rear_ear_v2_heatset (Autodesk Fusion 360 design; units mm, degrees)
part number: 2025-11-01-16-26-23-759
Autodesk Fusion 360 part; units mm, degrees
note: some values were not read from the file. Chosen so that the rebuilt part matches the saved one: a direction; which bodies a step acts on. Set by a fixed rule: which sketch regions a step uses.
sketch "Sketch1" plane through (0, 0, 0) normal (0, 0, 1) x (1, 0, 0)
  line L0 (0, 0) -> (15.875, 0)
  line L1 (15.875, 0) -> (15.875, 44.45)
  line L2 (15.875, 44.45) -> (0, 44.45)
  line L3 (0, 44.45) -> (0, 0)
  circle A0 centre (7.9375, 6.35) radius 2.4
  line L4 (7.9375, 44.45) -> (7.9375, 0) construction
  line L5 (0, 6.35) -> (15.875, 6.35) construction
  line L6 (0, 22.225) -> (15.875, 22.225) construction
  circle A1 centre (7.9375, 6.35) radius 2.4
  line L7 (15.875, 38.1) -> (0, 38.1) construction
  circle A2 centre (7.9375, 38.1) radius 2.4
  dimension "d1" = 15.875
  dimension "d2" = 44.45
  dimension "d5" = 6.35
  dimension "d6" = 15.875
  dimension "d7" = 4.8
  dimension "d9" = 15.875
  dimension "d10" = 4.8
  constraint horizontal L0
  constraint vertical L1
  constraint horizontal L2
  constraint vertical L3
  constraint coincident L0.start L3.end
  constraint midpoint L2 L4.start
  constraint midpoint L0 L4.end
  constraint coincident A0.centre L4
  constraint coincident L3 L5.start
  constraint coincident L1 L5.end
  constraint perpendicular L1 L5
  constraint midpoint A0.centre L5
  constraint coincident L3 L6.start
  constraint coincident L1 L6.end
  constraint perpendicular L1 L6
  constraint coincident L1 L7.start
  constraint coincident L3 L7.end
  constraint midpoint L7 A2.centre
  measures "d1" distance of L0.start L0.end
  measures "d2" distance of L0.start L2.end
  measures "d5" distance of L0 L5
  measures "d6" distance of L5 L6
  measures "d7" diameter of A1
  measures "d9" distance of L6 L7
  measures "d10" diameter of A2
extrude "Extrude1" add sketch "Sketch1" along normal blind 2 makes body 1
sketch "Sketch2" plane through (0, 0, 0) normal (-1, 0, 0) x (0, -1, 0)
  line L0 (-44.45, 0) -> (0, 0)
  line L1 (0, 0) -> (0, 2)
  line L2 (0, 2) -> (-44.45, 2)
  line L3 (-44.45, 2) -> (-44.45, 0)
  line L4 (-44.45, 0) -> (0, 0)
  line L5 (0, 0) -> (0, 65)
  line L6 (0, 65) -> (-44.45, 65)
  line L7 (-44.45, 65) -> (-44.45, 0)
  line L8 (-22.225, 0) -> (-22.225, 65) construction
  line L9 (-22.225, 65) -> (-10.225, 65)
  line L10 (-10.225, 65) -> (-10.225, 0)
  line L11 (-10.225, 0) -> (-22.225, 0)
  line L12 (-22.225, 0) -> (-22.225, 65)
  line L13 (-22.225, 65) -> (-34.225, 65)
  line L14 (-34.225, 65) -> (-34.225, 0)
  line L15 (-34.225, 0) -> (-22.225, 0)
  line L16 (-22.225, 0) -> (-22.225, 65)
  dimension "d13" = 65
  dimension "d14" = 12
  dimension "d15" = 12
  dimension "d59" = 10.225
  constraint horizontal L4
  constraint vertical L5
  constraint horizontal L6
  constraint vertical L7
  constraint coincident L0.start L3.end
  constraint midpoint L0 L8.start
  constraint midpoint L6 L8.end
  constraint horizontal L9
  constraint vertical L10
  constraint horizontal L11
  constraint vertical L12
  constraint horizontal L13
  constraint vertical L14
  constraint horizontal L15
  constraint vertical L16
  measures "d13" distance of L0.start L6.end
  measures "d14" distance of L8.end L9.end
  measures "d15" distance of L8.end L13.end
  measures "d59" distance of L7 L14
extrude "Extrude2" add sketch "Sketch2" along normal blind 15 contours L0 L2 L3 L4 L7 L14 | L2 L6 L7 L14 | L0 L1 L2 L4 L5 L10 | L2 L5 L6 L10 bodies 1
fillet "Outer Edge Fillet" radius 5 2 edges at (15.875, 0, 1) (15.875, 44.45, 1) on bodies 1
sketch "Sketch4" plane through (0, 0, 65) normal (0, 0, 1) x (-1, 0, 0)
  line L0 (0, -10.225) -> (15, -10.225)
  line L1 (7.5, -10.225) -> (7.5, -0.5) construction
  circle A0 centre (7.5, -6.225) radius 4
  line L2 (15, -10.225) -> (15, 0)
  line L3 (0, 0) -> (0, -10.225)
  line L4 (15, 0) -> (0, 0)
  line L5 (0, -34.225) -> (15, -34.225)
  line L6 (0, -44.45) -> (15, -44.45)
  line L7 (7.5, -34.225) -> (7.5, -44.45) construction
  circle A1 centre (7.5, -38.225) radius 4
  circle A2 centre (7.5, -6.225) radius 1
  circle A3 centre (7.5, -38.225) radius 1
  dimension "d37" = 8
  dimension "d41" = 8
  dimension "d42" = 2
  dimension "d43" = 2
  constraint midpoint L0 L1.start
  constraint coincident L1 A0.centre
  constraint tangent L0 A0
  constraint midpoint L5 L7.start
  constraint midpoint L6 L7.end
  constraint coincident L7 A1.centre
  constraint tangent L5 A1
  constraint concentric A0 A2
  constraint concentric A1 A3
  measures "d37" diameter of A0
  measures "d41" diameter of A1
  measures "d42" diameter of A2
  measures "d43" diameter of A3
sketch "Sketch6" plane through (0, 0, 65) normal (0, 0, 1) x (-1, 0, 0)
  line L0 (0, -34.225) -> (0, -44.45)
  line L1 (0, -44.45) -> (15, -44.45)
  line L2 (15, -44.45) -> (15, -34.225)
  line L3 (15, -34.225) -> (0, -34.225)
  line L4 (0, -44.45) -> (15, -44.45)
  line L5 (0, 0) -> (15, 0)
  line L6 (0, 0) -> (15, 0)
  line L7 (15, 0) -> (15, -44.45)
  line L8 (15, -44.45) -> (0, -44.45)
  line L9 (0, -44.45) -> (0, 0)
  constraint horizontal L6
  constraint vertical L7
  constraint horizontal L8
  constraint vertical L9
  constraint coincident L1.end L2.start
  constraint coincident L5.start L6.start
extrude "Back Plate" add sketch "Sketch6" along normal blind 2 separate body makes body 2
extrude "Rod Hole Cut" cut sketch "Sketch4" against normal up to surface (65 mm away) contours A0 | A1 | A2 | A3 bodies 1
sketch "Tangency relief" plane through (0, 0, 0) normal (0, 0, 1) x (1, 0, 0)
  line L0 (-12.5, 10.1) -> (-2.5, 10.1)
  line L1 (-2.5, 10.1) -> (-2.5, 34.35)
  line L2 (-2.5, 34.35) -> (-12.5, 34.35)
  line L3 (-12.5, 34.35) -> (-12.5, 10.1)
extrude "Tangency relief (1)" cut sketch "Tangency relief" along normal blind 67 bodies 1
sketch "Laptop clearance" plane through (0, 0, 0) normal (0, 0, 1) x (1, 0, 0)
  line L0 (-0.05, 9.7) -> (0.65, 9.7)
  line L1 (0.65, 9.7) -> (0.65, 34.7)
  line L2 (0.65, 34.7) -> (-0.05, 34.7)
  line L3 (-0.05, 34.7) -> (-0.05, 9.7)
extrude "Laptop clearance (1)" cut sketch "Laptop clearance" along normal blind 67 bodies 1 2
ref_plane "WorkPlane1" through (0, 0, 67) normal (0, 0, 1) x (1, 0, 0)
ref_plane "WorkPlane2" through (0, 0, 69) normal (0, 0, 1) x (1, 0, 0)
sketch "Insert pockets (1)" plane through (0, 0, 69) normal (0, 0, 1) x (1, 0, 0)
  circle A0 centre (-7.5, 15) radius 2
  circle A1 centre (-7.5, 29.45) radius 2
extrude "Insert pockets (2)" cut sketch "Insert pockets (1)" along normal mid plane 0.4 bodies 1
sketch "Side wall" plane through (0, 0, 0) normal (0, 0, 1) x (1, 0, 0)
  line L0 (0, 0) -> (2, 0)
  line L1 (2, 0) -> (2, 44.45)
  line L2 (2, 44.45) -> (0, 44.45)
  line L3 (0, 44.45) -> (0, 0)
extrude "Side wall (2)" add sketch "Side wall" along normal blind 69 bodies 1 2
sketch "Boss pad" plane through (0, 0, 67) normal (0, 0, 1) x (1, 0, 0)
  line L0 (0, 0) -> (2, 0)
  line L1 (2, 0) -> (2, 44.45)
  line L2 (2, 44.45) -> (0, 44.45)
  line L3 (-0.05, 34.7) -> (0, 34.7)
  line L4 (0, 44.45) -> (-15, 44.45)
  line L5 (-15, 44.45) -> (-15, 0)
  line L6 (-15, 0) -> (0, 0)
  line L7 (0, 9.7) -> (-0.05, 9.7)
  line L8 (-15, 44.45) -> (2, 44.45)
  line L9 (2, 44.45) -> (2, 0)
  line L10 (2, 0) -> (-15, 0)
  line L11 (-15, 0) -> (-15, 44.45)
  constraint horizontal L8
  constraint vertical L9
  constraint horizontal L10
  constraint vertical L11
  constraint coincident L0.end L1.start
  constraint coincident L4.end L5.start
extrude "Boss pad (1)" add sketch "Boss pad" along normal blind 3 bodies 1
sketch "Insert pockets" plane through (0, 0, 69) normal (0, 0, 1) x (1, 0, 0)
  circle A0 centre (-7.5, 15) radius 2
  circle A1 centre (-7.5, 29.45) radius 2
extrude "Extrude17" add 1 faces at (-9.3333, 29.6333, 70) along direction (0, 0, 1) blind 2 on bodies 1 bodies 1
sketch "Duct rail" plane through (0, 0, 0) normal (0, 0, 1) x (1, 0, 0)
  line L0 (-25, 0) -> (-15, 0)
  line L1 (-15, 0) -> (-15, 6.4)
  line L2 (-15, 6.4) -> (-25, 6.4)
  line L3 (-25, 6.4) -> (-25, 0)
  line L4 (-25, 38.05) -> (-15, 38.05)
  line L5 (-15, 38.05) -> (-15, 44.45)
  line L6 (-15, 44.45) -> (-25, 44.45)
  line L7 (-25, 44.45) -> (-25, 38.05)
extrude "Duct rail (1)" add sketch "Duct rail" along normal blind 72 bodies 1
sketch "Duct panel slot" plane through (0, 0, 0) normal (0, 0, 1) x (1, 0, 0)
  line L0 (-25.1, 2) -> (-13, 2)
  line L1 (-13, 2) -> (-13, 4.4)
  line L2 (-13, 4.4) -> (-25.1, 4.4)
  line L3 (-25.1, 4.4) -> (-25.1, 2)
  line L4 (-25.1, 40.05) -> (-13, 40.05)
  line L5 (-13, 40.05) -> (-13, 42.45)
  line L6 (-13, 42.45) -> (-25.1, 42.45)
  line L7 (-25.1, 42.45) -> (-25.1, 40.05)
extrude "Duct panel slot (1)" cut sketch "Duct panel slot" along normal through all bodies 1
ref_plane "WorkPlane3" through (0, 0, 68.8) normal (0, 0, 1) x (1, 0, 0)
sketch "Insert pocket bore" plane through (0, 0, 68.8) normal (0, 0, 1) x (1, 0, 0)
  circle A0 centre (-7.5, 15) radius 2
  circle A1 centre (-7.5, 29.45) radius 2
extrude "Insert pocket bore (1)" cut sketch "Insert pocket bore" along normal blind 3.4 bodies 1
sketch "Laptop relief recut" plane through (0, 0, 0) normal (0, 0, 1) x (1, 0, 0)
  line L0 (-0.05, 9.7) -> (0.65, 9.7)
  line L1 (0.65, 9.7) -> (0.65, 34.7)
  line L2 (0.65, 34.7) -> (-0.05, 34.7)
  line L3 (-0.05, 34.7) -> (-0.05, 9.7)
extrude "Laptop relief recut (1)" cut sketch "Laptop relief recut" along normal blind 67.1 bodies 1
equation "d1 = bracket_width"
equation "d2 = ru"
equation "d5 = ru_gap"
equation "d6 = hole_spacing"
equation "d7 = hole_diameter"
equation "d9 = hole_spacing"
equation "d10 = hole_diameter"
equation "d11 = thickness"
equation "d13 = rear_depth"
equation "d14 = laptop_thickness / 2"
equation "d15 = laptop_thickness / 2"
equation "d16 = ear_width"
equation "thickness = 2 mm"
equation "laptop_thickness = 24 mm"
equation "hole_diameter = 4.8 mm"
equation "ru_gap = 6.35 mm"
equation "hole_spacing = 15.875 mm"
equation "ru = 44.45 mm"
equation "bracket_width = 15.875 mm"
equation "ear_width = 15 mm"
equation "rod_diameter = 8 mm"
equation "rear_depth = 65 mm"
equation "d37 = rod_diameter"
equation "front_depth = 6 mm"
equation "d41 = rod_diameter"
equation "d56 = thickness"
equation "d67 = rear_depth + thickness"
equation "d71 = rear_depth + ( 2 * thickness )"
equation "d73 = insert_pocket_relief"
equation "d75 = rear_depth + ( 2 * thickness )"
equation "d81 = thickness"
equation "duct_rail_length = 10.00 mm" comment "rail reach toward the rack centre"
equation "duct_slot_height = 2.40 mm" comment "panel thickness plus running clearance"
equation "duct_wall = 2.00 mm" comment "wall either side of the panel slot"
equation "duct_groove_depth = 2.00 mm" comment "pocket cut into the ear inner face"
equation "insert_pocket_relief = 0.4 mm" comment "full length of the symmetric relief under the boss pad"
named bodies: "Rear Ear", "Back Plate"
